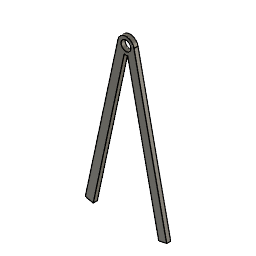
00_FULL-ASSEMBLY (Autodesk Fusion 360 archive; units mm, degrees)
design "servo arm"
Autodesk Fusion 360 part; units mm, degrees
sketch "Sketch1" plane through (0, 0, 0) normal (0, 1, 0) x (1, 0, 0)
  circle A0 centre (0, 0) radius 3
  line L0 (0, 0) -> (0, 93.3) construction
  line L1 (0, 93.3) -> (-20, 93.3) construction
  line L2 (-0.9432, 4.4) -> (-20, 93.3)
  line L3 (-20, 93.3) -> (-24.8889, 92.252)
  line L4 (-24.8889, 92.252) -> (-4.8889, -1.048)
  line L5 (-20, 93.3) -> (-0.9432, 4.4) construction
  line L6 (-0.6288, 2.9334) -> (0, 0) construction
  line L7 (24.8889, 92.252) -> (4.8889, -1.048)
  line L8 (1.048, 4.8889) -> (0.9432, 4.4) construction
  line L9 (20, 93.3) -> (24.8889, 92.252)
  line L10 (20, 93.3) -> (0.9432, 4.4)
  arc A1 (-4.8889, -1.048) -> (4.8889, -1.048) centre (0, 0) ccw
  arc A2 (1.048, 4.8889) -> (-1.048, 4.8889) centre (0, 0) ccw
  dimension "d1" = 6
  dimension "d2" = 93.3
  dimension "d3" = 20
  dimension "d5" = 5
  dimension "d6" = 10
  constraint coincident A0.centre L0.start
  constraint vertical L0
  constraint perpendicular L0 L1
  constraint perpendicular L2 L3
  constraint perpendicular L3 L4
  constraint coincident A0 L6.start
  constraint collinear L5 L6
  constraint concentric A0 A1
  constraint symmetric L0 L1.end L9.start
  constraint symmetric L0 L2.start L8.end
  constraint symmetric L0 L3.end L7.start
  constraint symmetric L0 L4.end L7.end
  constraint coincident L2 A2.end
  constraint concentric A1 A2
  measures "d1" diameter of A0
  measures "d2" distance of A0.centre L0.end
  measures "d3" distance of L0.end L1.end
  measures "d5" distance of L1.end L3.end
  measures "d6" diameter of A1
extrude "Extrude1" add sketch "Sketch1" along normal blind 2.5
